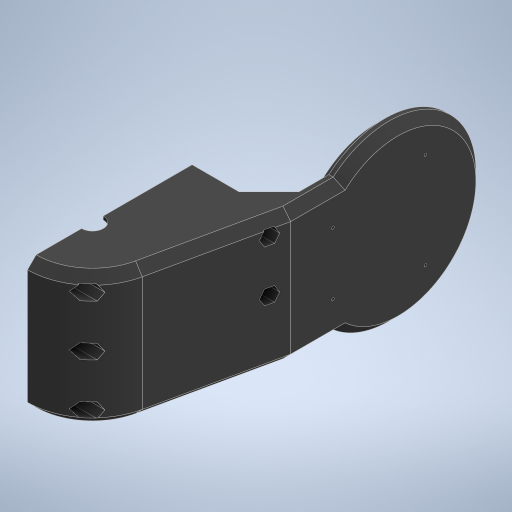
# Autodesk Inventor part: Wirst_2L
Saved by Autodesk Inventor 2023 (Build 270158000, 158)
## iProperties
Created: 2024-07-25
Part Number: Wirst_2L
Material: Generic
Document SubType Name: Modeling
Designer: Swoby
Density: 1 g/cm^3
Appearance: Default
Author: Swoby
Autodesk Inventor part; units mm, degrees
ref_plane "YZ Plane" through (0, 0, 0) normal (1, 0, 0) x (0, 1, 0)
ref_plane "XZ Plane" through (0, 0, 0) normal (0, 1, 0) x (-1, 0, 0)
ref_plane "XY Plane" through (0, 0, 0) normal (0, 0, 1) x (1, 0, 0)
sketch "Sketch1" plane through (0, 0, 0) normal (0, 1, 0) x (-1, 0, 0)
  arc A0 (0, -30) -> (0, 30) centre (0, 0) ccw
  line L0 (29.3229, 6.338) -> (41.5, -50)
  line L1 (0, 30) -> (0, -50)
  line L2 (0, -50) -> (20, -50)
  line L3 (20, -50) -> (31.5, -61.5)
  line L4 (31.5, -61.5) -> (31.5, -101.5)
  line L5 (31.5, -101.5) -> (41.5, -101.5)
  line L6 (41.5, -101.5) -> (41.5, -50)
  dimension "d0" = 60
  dimension "d1" = 31.5
  dimension "d2" = 10
  dimension "d3" = 50
  dimension "d7" = 135
  dimension "d8" = 20
  dimension "d9" = 40
  constraints: 14 end point, 3 perpendicular, 3 point on circle, 3 point on line, 1 centre point, 1 coincident, 1 horizontal, 1 tangent, 1 vertical
  measures "d0" diameter of A0
  measures "d1" distance between parallel lines of L1 L4
  measures "d2" distance between parallel lines of L4 L6
  measures "d3" distance from line of point (0, 0) L2
  measures "d7" angle of L2 L3
  measures "d8" distance of L1.end L2.end
  measures "d9" distance of L3.end L4.end
extrude "Extrusion1" add sketch "Sketch1" along normal mid plane 61
sketch "Sketch2" plane through (0, -30.5, -50) normal (1, 0, 0) x (0, 0, -1)
  line L0 (-60.65, 57.9) -> (-50, 57.9)
  line L1 (-19.05, 57.9) -> (-19.05, 50.4)
  line L2 (-19.05, 17.3) -> (-60.65, 17.3)
  line L3 (-60.65, 17.3) -> (-60.65, 46.7)
  line L4 (-60.65, 50.4) -> (-67.75, 50.4)
  line L5 (-67.75, 50.4) -> (-67.75, 46.7)
  line L6 (-67.75, 46.7) -> (-60.65, 46.7)
  line L7 (-19.05, 46.7) -> (-11.95, 46.7)
  line L8 (-11.95, 46.7) -> (-11.95, 50.4)
  line L9 (-11.95, 50.4) -> (-19.05, 50.4)
  line L10 (-19.05, 26.6) -> (-11.95, 26.6)
  line L11 (-11.95, 26.6) -> (-11.95, 21.2)
  line L12 (-11.95, 21.2) -> (-19.05, 21.2)
  line L13 (-60.65, 50.4) -> (-60.65, 57.9)
  line L14 (-19.05, 46.7) -> (-19.05, 26.6)
  line L15 (-19.05, 21.2) -> (-19.05, 17.3)
  line L16 (-50, 61) -> (-50, 0)
  line L17 (-80, 0) -> (-80, 61) projected
  line L18 (-57.4, 59.4) -> (-50, 59.4)
  line L19 (-43.05, 57.9) -> (-57.4, 57.9)
  line L20 (-57.4, 57.9) -> (-57.4, 59.4)
  line L21 (-55, 61) -> (-50, 61)
  line L22 (-55, 45.4) -> (-55, 61)
  line L23 (-50, 0) -> (-62.4, 0)
  line L24 (-62.4, 0) -> (-62.4, 5.5)
  line L25 (-62.4, 5.5) -> (-50, 5.5)
  line L26 (-50, 5.5) -> (-50, 0)
  line L27 (0, 0) -> (-80, 0) projected
  line L28 (-50, 57.9) -> (-19.05, 57.9)
  line L29 (-50, 54) -> (-50, 57.9)
  line L30 (-80, 61) -> (0, 61) projected
  point P0 (-50, 30.5)
  point P1 (-64.2, 46.7)
  point P2 (-64.2, 50.4)
  point P3 (-55, 53.2)
  point P4 (-55, 59.4)
  point P5 (-57.4, 57.9)
  point P6 (-50, 50.9)
  point P7 (-50, 5.5)
  dimension "d12" = 41.6
  dimension "d13" = 40.6
  dimension "d15" = 7.1
  dimension "d16" = 7.5
  dimension "d17" = 3.7
  dimension "d18" = 30
  dimension "d20" = 10.65
  dimension "d22" = 7.1
  dimension "d23" = 3.9
  dimension "d24" = 5.4
  dimension "d27" = 7.4
  dimension "d28" = 5
  dimension "d32" = 5.5
  dimension "d33" = 12.4
  dimension "d34" = 1.6
  dimension "d35" = 1.5
  dimension "d36" = 3.1
  constraints: 56 end point, 14 perpendicular, 14 point on line, 12 parallel, 7 horizontal, 3 collinear, 3 midpoint, 2 vertical, 1 other
  measures "d12" distance of L0.start L1.start
  measures "d13" distance between parallel lines of L2 L0
  measures "d15" distance of L4.start L4.end
  measures "d16" distance between parallel lines of L0 L4
  measures "d17" distance of point (-64.2, 46.7) point (-64.2, 50.4)
  measures "d18" distance between parallel lines of L17 L16
  measures "d20" distance between parallel lines of L16 L3
  measures "d22" distance of L8.end L1.end
  measures "d23" distance of L12.end L2.start
  measures "d24" distance of L10.end L11.end
  measures "d27" distance between parallel lines of L20 L16
  measures "d28" distance from line of L16 point (-55, 53.2)
  measures "d32" distance of L23.end L24.end
  measures "d33" distance of L24.end L25.end
  measures "d34" distance between parallel lines of L18 L21
  measures "d35" distance between parallel lines of L19 L18
extrude "Extrusion2" cut sketch "Sketch2" against normal blind 11.3 contours L0 L16 L2 L3 L6 L5 L4 L13 | L19 L28 L1 L9 L8 L7 L14 L10 L11 L12 L15 L2 L16
revolve "Revolution1" cut sketch "Sketch2" angle 360 about axis through (0, 30.5, 0) along (0, 1, 0) contours L20 L18 L22 L0 | L22 L18 L16 L0 | L22 L21 L16 L18 | L16 L23 L24 L25
sketch "Sketch3" plane through (0, -30.5, -50) normal (1, 0, 0) x (0, 0, -1)
  line L0 (-62.4, 0) -> (-62.4, 5.5) projected
  line L1 (-37.6, 0) -> (-62.4, 0) projected
  line L2 (-37.6, 5.5) -> (-37.6, 0) projected
  line L3 (-37.6, 5.5) -> (-62.4, 5.5) projected
  line L4 (-62.4, 5.5) -> (-50, 13.3)
  line L5 (-50, 13.3) -> (-16.9, 13.3)
  line L6 (-50, 5.5) -> (-50, 0)
  line L7 (-19.05, 17.3) -> (-60.65, 17.3) projected
  line L8 (-37.6, 7.3) -> (-16.9, 7.3)
  line L9 (-11.95, 21.2) -> (-19.05, 21.2) projected
  line L10 (-67.75, 46.7) -> (-67.75, 50.4) projected
  line L11 (-60.65, 46.7) -> (-67.75, 46.7) projected
  line L12 (-60.65, 17.3) -> (-60.65, 46.7) projected
  line L13 (-19.05, 17.3) -> (-60.65, 17.3) projected
  line L14 (-19.05, 21.2) -> (-19.05, 17.3) projected
  line L15 (-11.95, 21.2) -> (-19.05, 21.2) projected
  line L16 (-11.95, 26.6) -> (-11.95, 21.2) projected
  line L17 (-19.05, 26.6) -> (-11.95, 26.6) projected
  line L18 (-19.05, 46.7) -> (-19.05, 26.6) projected
  line L19 (-11.95, 46.7) -> (-19.05, 46.7) projected
  line L20 (-11.95, 50.4) -> (-11.95, 46.7) projected
  line L21 (-19.05, 50.4) -> (-11.95, 50.4) projected
  line L22 (-19.05, 57.9) -> (-19.05, 50.4) projected
  line L23 (-60.65, 57.9) -> (-19.05, 57.9) projected
  line L24 (-60.65, 50.4) -> (-60.65, 57.9) projected
  line L25 (-67.75, 50.4) -> (-60.65, 50.4) projected
  line L26 (-11.95, 26.6) -> (-3, 26.6)
  line L27 (-3, 26.6) -> (-3, 21.2)
  line L28 (-9, 21.2) -> (-11.95, 21.2)
  arc A0 (-16.9, 7.3) -> (-3, 21.2) centre (-16.9, 21.2) ccw
  arc A1 (-16.9, 13.3) -> (-9, 21.2) centre (-16.9, 21.2) ccw
  line L29 (0, 0) -> (0, 61) projected
  line L30 (-37.6, 5.5) -> (-37.6, 7.3)
  point P0 (-50, 30.5)
  dimension "d37" = 4
  dimension "d46" = 3
  dimension "d48" = 13.9
  dimension "d49" = 13.9
  dimension "d52" = 6
  constraints: 16 end point, 4 point on circle, 3 tangent, 2 centre point, 2 horizontal, 2 midpoint, 2 perpendicular, 2 point on line, 1 collinear, 1 concentric
  measures "d37" distance between parallel lines of L5 L7
  measures "d46" distance between parallel lines of L29 L27
  measures "d48" distance between parallel lines of L8 L28
  measures "d49" radius of A0
  measures "d52" distance between parallel lines of L8 L5
extrude "Extrusion3" cut sketch "Sketch3" against normal up to surface (11.3 mm away) contours L4 L5 A1 L28 L16 L26 L27 A0 L8 L30 L3
sketch "Sketch5" plane through (-31.5, -30.5, -101.5) normal (1, 0, 0) x (0, 0, -1)
  line L0 (0, 0) -> (0, 61) projected
  line L1 (-40, 0) -> (-40, 61) projected
  line L2 (0, 30.5) -> (-40, 30.5) construction
  circle A0 centre (-2, 30.5) radius 40
  point P0 (-101.5, 30.5)
  point P1 (-40, 42.99)
  point P2 (-40, 18.01)
  dimension "d63" = 80
  dimension "d64" = 38
  constraints: 2 end point, 2 midpoint, 1 centre point, 1 perpendicular, 1 point on line
  measures "d63" diameter of A0
  measures "d64" distance from line of L1 A0.centre
extrude "Extrusion5" add sketch "Sketch5" against normal up to surface (10 mm away) contours L1 A0 picked at (8.4702, 47.4774)
chamfer "Chamfer3" distance 4 angle 45 14 edges at (-18.8396, 30.5, 23.3467) (-35.4114, 30.5, -21.831) (-41.5, 30.5, -61.8102) (-41.5, 0, -139.5) (-41.5, -30.5, -61.8102) (-35.4114, -30.5, -21.831) (-18.8396, -30.5, 23.3467) (-31.5, 0, -139.5) (-25.75, 30.5, -55.75) (-31.5, 30.5, -67.5602) (-10, 30.5, -50) (-10, -30.5, -50) (-25.75, -30.5, -55.75) (-31.5, -30.5, -67.5602)
sketch "Sketch9" plane through (0, -13.2, 10.65) normal (1, 0, 0) x (0, 0, -1)
  circle A0 centre (-11.35, 36.7) radius 2
  circle A1 centre (-11.35, -10.3) radius 2
  circle A2 centre (52.65, 36.7) radius 2
  circle A3 centre (52.65, 13.2) radius 2
  circle A4 centre (-11.35, 13.2) radius 2
  line L0 (-19.35, 39.7) -> (-15.35, 43.7) projected
  line L1 (-19.35, -13.3) -> (-19.35, 39.7) projected
  line L2 (-15.35, -17.3) -> (-19.35, -13.3) projected
  line L3 (-1.75, -17.3) -> (-15.35, -17.3) projected
  line L4 (-1.75, -17.3) -> (-1.75, -11.8) projected
  line L5 (-1.75, -11.8) -> (10.65, -4) projected
  line L6 (10.65, -4) -> (43.75, -4) projected
  arc A5 (43.75, -4) -> (51.65, 3.9) centre (43.75, 3.9) ccw projected
  line L7 (51.65, 3.9) -> (41.6, 3.9) projected
  line L8 (41.6, 3.9) -> (41.6, 0) projected
  line L9 (41.6, 0) -> (0, 0) projected
  line L10 (0, 0) -> (0, 29.4) projected
  line L11 (0, 29.4) -> (-7.1, 29.4) projected
  line L12 (-7.1, 29.4) -> (-7.1, 33.1) projected
  line L13 (-7.1, 33.1) -> (0, 33.1) projected
  line L14 (0, 33.1) -> (0, 40.6) projected
  line L15 (0, 40.6) -> (3.25, 40.6) projected
  line L16 (3.25, 40.6) -> (3.25, 42.1) projected
  line L17 (3.25, 42.1) -> (5.65, 42.1) projected
  line L18 (5.65, 42.1) -> (5.65, 43.7) projected
  line L19 (-15.35, 43.7) -> (5.65, 43.7) projected
  line L20 (60.65, -13.3) -> (56.65, -17.3) projected
  line L21 (60.65, -13.3) -> (60.65, 39.7) projected
  line L22 (56.65, 43.7) -> (60.65, 39.7) projected
  line L23 (15.65, 43.7) -> (56.65, 43.7) projected
  line L24 (15.65, 43.7) -> (15.65, 42.1) projected
  line L25 (15.65, 42.1) -> (18.05, 42.1) projected
  line L26 (18.05, 42.1) -> (18.05, 40.6) projected
  line L27 (18.05, 40.6) -> (41.6, 40.6) projected
  line L28 (41.6, 40.6) -> (41.6, 33.1) projected
  line L29 (41.6, 33.1) -> (48.7, 33.1) projected
  line L30 (48.7, 33.1) -> (48.7, 29.4) projected
  line L31 (48.7, 29.4) -> (41.6, 29.4) projected
  line L32 (41.6, 29.4) -> (41.6, 9.3) projected
  line L33 (41.6, 9.3) -> (57.65, 9.3) projected
  line L34 (57.65, 9.3) -> (57.65, 3.9) projected
  arc A6 (43.75, -10) -> (57.65, 3.9) centre (43.75, 3.9) ccw projected
  line L35 (43.75, -10) -> (23.05, -10) projected
  line L36 (56.65, -17.3) -> (23.05, -17.3) projected
  line L37 (-11.35, 13.2) -> (52.65, 13.2) construction
  line L38 (23.05, -10) -> (23.05, -11.8) projected
  line L39 (23.05, -11.8) -> (23.05, -17.3) projected
  line L40 (-19.35, 39.7) -> (-15.35, 43.7) projected
  line L41 (-19.35, -13.3) -> (-19.35, 39.7) projected
  line L42 (-15.35, -17.3) -> (-19.35, -13.3) projected
  line L43 (-1.75, -17.3) -> (-15.35, -17.3) projected
  line L44 (-1.75, -17.3) -> (-1.75, -11.8) projected
  line L45 (-1.75, -11.8) -> (10.65, -4) projected
  line L46 (10.65, -4) -> (43.75, -4) projected
  arc A7 (43.75, -4) -> (51.65, 3.9) centre (43.75, 3.9) ccw projected
  line L47 (51.65, 3.9) -> (41.6, 3.9) projected
  line L48 (41.6, 3.9) -> (41.6, 0) projected
  line L49 (41.6, 0) -> (0, 0) projected
  line L50 (0, 0) -> (0, 29.4) projected
  line L51 (0, 29.4) -> (-7.1, 29.4) projected
  line L52 (-7.1, 29.4) -> (-7.1, 33.1) projected
  line L53 (-7.1, 33.1) -> (0, 33.1) projected
  line L54 (0, 33.1) -> (0, 40.6) projected
  line L55 (0, 40.6) -> (3.25, 40.6) projected
  line L56 (3.25, 40.6) -> (3.25, 42.1) projected
  line L57 (3.25, 42.1) -> (5.65, 42.1) projected
  line L58 (5.65, 42.1) -> (5.65, 43.7) projected
  line L59 (-15.35, 43.7) -> (5.65, 43.7) projected
  point P0 (60.65, 11.8)
  point P1 (-19.35, 13.2)
  point P2 (60.65, 13.2)
  dimension "d92" = 4
  dimension "d103" = 4
  dimension "d120" = 8
  dimension "d127" = 7
  dimension "d128" = 8
  dimension "d129" = 8
  dimension "d131" = 8
  dimension "d132" = 7
  dimension "d133" = 4
  dimension "d134" = 4
  dimension "d135" = 4
  dimension "d136" = 7
  dimension "d137" = 8
  dimension "d138" = 8
  constraints: 5 centre point, 2 end point, 2 midpoint, 1 coincident, 1 horizontal, 1 point on line
  measures "d92" diameter of A3
  measures "d103" diameter of A4
  measures "d120" horizontal distance of point (60.65, 11.8) L37.end
  measures "d127" distance from line of L19 point (-11.35, 36.7)
  measures "d128" distance from line of L1 A0.centre
  measures "d129" distance from line of L1 A1.centre
  measures "d131" distance from line of L21 A2.centre
  measures "d132" distance from line of L3 A1.centre
  measures "d133" diameter of A0
  measures "d134" diameter of A1
  measures "d135" diameter of A2
  measures "d136" distance from line of L23 A2.centre
  measures "d137" distance from line of L1 L37.start
  measures "d138" distance of point (60.65, 13.2) L37.end
extrude "Extrusion9" cut sketch "Sketch9" against normal through all contours A0 | A1 | A2 | A3 | A4
chamfer "Chamfer5" distance 1.75 angle 45 1 edges at (-5.65, -23.2, -12.4)
mirror "Mirror1" about plane through (0, 0, 30) normal (1, 0, 0) remove original yes
ref_plane "Work Plane2" through (6, -26.5, -50) normal (-1, 0, 0) x (0, 0, 1)
sketch "Sketch12" plane through (6, -26.5, -50) normal (-1, 0, 0) x (0, 0, 1)
  circle A0 centre (8, 26.5) radius 2 projected
  circle A1 centre (8, 50) radius 2 projected
  circle A2 centre (72, 3) radius 2 projected
  circle A3 centre (72, 26.5) radius 2 projected
  circle A4 centre (72, 50) radius 2 projected
  line L0 (70.0659, 6.35) -> (73.9341, 6.35)
  line L1 (73.9341, 6.35) -> (75.8682, 3)
  line L2 (75.8682, 3) -> (73.9341, -0.35)
  line L3 (73.9341, -0.35) -> (70.0659, -0.35)
  line L4 (70.0659, -0.35) -> (68.1318, 3)
  line L5 (68.1318, 3) -> (70.0659, 6.35)
  line L6 (70.0659, 29.85) -> (73.9341, 29.85)
  line L7 (73.9341, 29.85) -> (75.8682, 26.5)
  line L8 (75.8682, 26.5) -> (73.9341, 23.15)
  line L9 (73.9341, 23.15) -> (70.0659, 23.15)
  line L10 (70.0659, 23.15) -> (68.1318, 26.5)
  line L11 (68.1318, 26.5) -> (70.0659, 29.85)
  line L12 (70.0659, 53.35) -> (73.9341, 53.35)
  line L13 (73.9341, 53.35) -> (75.8682, 50)
  line L14 (75.8682, 50) -> (73.9341, 46.65)
  line L15 (73.9341, 46.65) -> (70.0659, 46.65)
  line L16 (70.0659, 46.65) -> (68.1318, 50)
  line L17 (68.1318, 50) -> (70.0659, 53.35)
  line L18 (4.1318, 50) -> (6.0659, 53.35)
  line L19 (6.0659, 53.35) -> (9.9341, 53.35)
  line L20 (9.9341, 53.35) -> (11.8682, 50)
  line L21 (11.8682, 50) -> (9.9341, 46.65)
  line L22 (9.9341, 46.65) -> (6.0659, 46.65)
  line L23 (6.0659, 46.65) -> (4.1318, 50)
  line L24 (6.0659, 29.85) -> (9.9341, 29.85)
  line L25 (9.9341, 29.85) -> (11.8682, 26.5)
  line L26 (11.8682, 26.5) -> (9.9341, 23.15)
  line L27 (9.9341, 23.15) -> (6.0659, 23.15)
  line L28 (6.0659, 23.15) -> (4.1318, 26.5)
  line L29 (4.1318, 26.5) -> (6.0659, 29.85)
  line L30 (76, 57) -> (55.4929, 57) projected
  line L31 (55.4929, 57) -> (-0.4274, 57) projected
  point P0 (50, 26.5)
  point P1 (72, 6.35)
  point P2 (72, -0.35)
  point P3 (72, 29.85)
  point P4 (72, 53.35)
  point P5 (72, 46.65)
  dimension "d153" = 6.7
  dimension "d154" = 6.7
  dimension "d155" = 6.7
  dimension "d156" = 6.7
  dimension "d157" = 6.7
  constraints: 60 end point, 5 coincident, 5 midpoint, 5 parallel, 65 other
  measures "d153" distance between parallel lines of L24 L27
  measures "d154" distance between parallel lines of L19 L22
  measures "d155" distance of point (72, 6.35) point (72, -0.35)
  measures "d156" distance from line of point (72, 29.85) L9
  measures "d157" distance of point (72, 53.35) point (72, 46.65)
extrude "Extrusion12" cut sketch "Sketch12" against normal through all
sketch "Sketch13" plane through (41.5, 0, -99.5) normal (1, 0, 0) x (0, 0, -1)
  line L0 (-30, 14.3) -> (-30, -14.3) construction
  line L1 (-30, -14.3) -> (12.75, -22.0835) construction
  line L2 (12.75, -22.0835) -> (12.75, 22.0835) construction
  line L3 (12.75, 22.0835) -> (-30, 14.3) construction
  arc A0 (-24.367, -26.5) -> (-24.367, 26.5) centre (0, 0) ccw projected
  line L4 (-49.5, -26.5) -> (-49.5, 26.5) projected
  circle A1 centre (-30, 14.3) radius 0.65
  circle A2 centre (-30, -14.3) radius 0.65
  circle A3 centre (12.75, -22.0835) radius 0.65
  circle A4 centre (12.75, 22.0835) radius 0.65
  point P0 (-99.5, 0)
  point P1 (-30, 0)
  dimension "d160" = 30
  dimension "d161" = 12.75
  dimension "d163" = 14.3
  dimension "d164" = 14.3
  dimension "d165" = 22.0835
  dimension "d166" = 22.0835
  dimension "d167" = 1.3
  dimension "d168" = 1.3
  dimension "d169" = 1.3
  dimension "d170" = 1.3
  constraints: 8 end point, 4 centre point, 4 coincident, 2 parallel, 1 midpoint, 1 vertical
  measures "d160" distance from line of A0.centre L0
  measures "d161" distance from line of L2 A0.centre
  measures "d163" vertical distance of L0.start A0.centre
  measures "d164" vertical distance of L0.end A0.centre
  measures "d165" vertical distance of L2.end A0.centre
  measures "d166" vertical distance of L1.end A0.centre
  measures "d167" diameter of A1
  measures "d168" diameter of A2
  measures "d169" diameter of A3
  measures "d170" diameter of A4
extrude "Extrusion13" cut sketch "Sketch13" against normal blind 5
equation "\"d22\" = d15"
equation "\"d49\" = d48"
equation "\"d120\" = d128"
equation "\"d129\" = d128"
equation "\"d131\" = d128"
equation "\"d132\" = d127"
body "Solid1"
